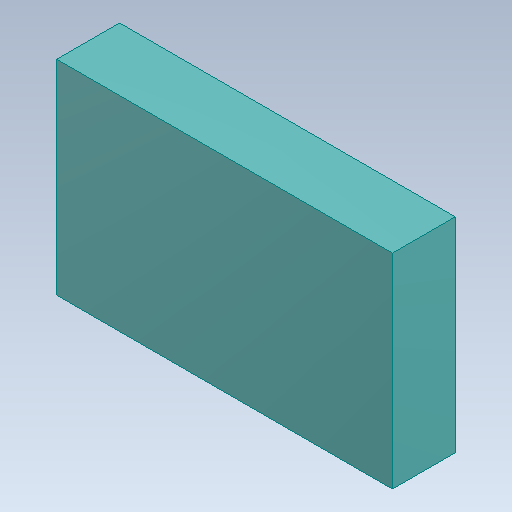
# Autodesk Inventor part: 47UF
Saved by Autodesk Inventor 2020 (Build 240168000, 168)
## iProperties
Created: 2019-08-29
Part Number: 47UF
Material: Generic
Document SubType Name: Modeling
Designer: psrob
Density: 1 g/cm^3
Appearance: EIA3528, 47UF
Author: psrob
Autodesk Inventor part; units mm, degrees
ref_plane "YZ Plane" through (0, 0, 0) normal (1, 0, 0) x (0, 1, 0)
ref_plane "XZ Plane" through (0, 0, 0) normal (0, 1, 0) x (-1, 0, 0)
ref_plane "XY Plane" through (0, 0, 0) normal (0, 0, 1) x (1, 0, 0)
sketch "EIA3528, 47UF_3" plane through (0, 0, 0) normal (0, 0, 1) x (1, 0, 0)
  line L0 (-2.7016, 1.55) -> (2.641, 1.55)
  line L1 (2.641, 1.55) -> (2.641, -1.7016)
  line L2 (2.641, -1.7016) -> (-2.7016, -1.7016)
  line L3 (-2.7016, -1.7016) -> (-2.7016, 1.55)
  constraints: 8 end point
extrude "Extrusion1" add sketch "EIA3528, 47UF_3" along normal blind 1
body "Solid1"
